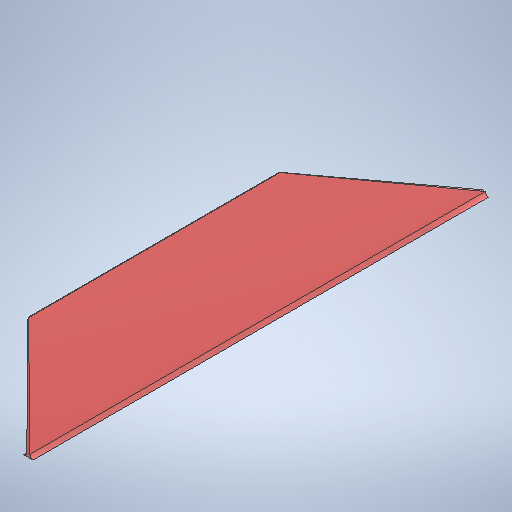
# Autodesk Inventor part: ALETAS
Saved by Autodesk Inventor 2025 (Build 290162000, 162)
## iProperties
Created: 2024-07-26
Part Number: ALETAS
Material: Generic
Document SubType Name: Modeling
Designer: Richard
Density: 1 g/cm^3
Appearance: Default
Author: Richard
Autodesk Inventor part; units mm, degrees
ref_plane "YZ Plane" through (0, 0, 0) normal (1, 0, 0) x (0, 1, 0)
ref_plane "XZ Plane" through (0, 0, 0) normal (0, 1, 0) x (-1, 0, 0)
ref_plane "XY Plane" through (0, 0, 0) normal (0, 0, 1) x (1, 0, 0)
sketch "Sketch1" plane through (0, 0, 0) normal (0, 0, 1) x (1, 0, 0)
  line L0 (-0.0053, 77.8701) -> (0.4947, 77.8701)
  line L1 (0.4947, 77.8701) -> (-0.5053, 77.8701)
  arc A0 (0.4947, 39.0706) -> (1.5528, 37.9683) centre (1.5979, 39.0706) ccw
  arc A1 (-1.5635, 37.9683) -> (-0.5053, 39.0714) centre (-1.6216, 39.0831) ccw
  line L2 (0.4947, 77.8701) -> (0.4947, 39.0706)
  line L3 (-0.5053, 77.8701) -> (-0.5053, 39.0714)
  arc A2 (1.5528, 37.9683) -> (-1.5635, 37.9683) centre (-0.0053, -38.0158) ccw
  line L4 (-0.0053, 77.8701) -> (0.0947, 77.8701)
  line L5 (-0.0053, 76.9579) -> (-0.0053, 77.45)
  line L6 (0.4947, 77.8701) -> (0.4947, 39.0706)
  line L7 (0.4947, 39.0706) -> (0.0947, 77.8701)
  line L8 (0, 77.8701) -> (-0.1, 77.8701)
  line L9 (-0.1, 77.8701) -> (-0.5053, 39.0714)
  point P0 (0, 0)
  dimension "d2" = 0.5
  dimension "d3" = 1
  dimension "d7" = 76
  dimension "d9" = 0.1
  dimension "d11" = 0.1
  constraints: 20 end point, 6 point on circle, 5 point on line, 3 centre point, 3 tangent, 2 vertical, 1 horizontal, 1 perpendicular
  measures "d2" distance of L0.start L0.end
  measures "d3" distance of L0.end L1.end
  measures "d7" radius of A2
  measures "d9" distance of L0.start L4.end
  measures "d11" distance of L8.start L8.end
extrude "Extrusion1" add sketch "Sketch1" along normal blind 150 contours L0 L7 A0 A2 A1 L9 L1
sketch "Sketch2" plane through (0.0947, 77.8701, 150) normal (0.9999469, 0.0103089, 0) x (0, 0, -1)
  line L0 (150, -38.8016) -> (43.624, 22.6146)
  line L1 (150, -38.8016) -> (272.8324, -38.8016) construction
  line L2 (150, 0) -> (150, -38.8016)
  line L3 (150, -38.8016) -> (150, 6.7888)
  line L4 (150, 6.7888) -> (63.7901, 6.7888)
  point P0 (150, -77.865)
  point P1 (71.0352, 6.7888)
  dimension "d14" = 150
  constraints: 10 end point, 2 horizontal, 1 equal length, 1 vertical
  measures "d14" angle of L1 L0
extrude "Extrusion2" cut sketch "Sketch2" against normal through all
body "Solid1"
